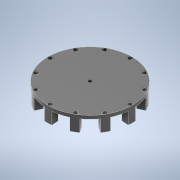
# Autodesk Inventor part: Platform
Saved by Autodesk Inventor 2022 (Build 260153000, 153)
## iProperties
Created: 2022-02-20
Part Number: Platform
Material: Genérico
Document SubType Name: Modeling
Designer: JK
Density: 1 g/cm^3
Appearance: Suave - Negro
Author: JK
Autodesk Inventor part; units mm, degrees
ref_plane "YZ Plane" through (0, 0, 0) normal (1, 0, 0) x (0, 1, 0)
ref_plane "XZ Plane" through (0, 0, 0) normal (0, 1, 0) x (-1, 0, 0)
ref_plane "XY Plane" through (0, 0, 0) normal (0, 0, 1) x (1, 0, 0)
sketch "Boceto1" plane through (0, 0, 0) normal (0, 1, 0) x (-1, 0, 0)
  circle A0 centre (0, 0) radius 62.862
  circle A1 centre (0, 0) radius 52.5
  dimension "d0" = 125.724
  dimension "d1" = 105
  constraints: 2 centre point, 2 coincident
  measures "d0" diameter of A0
  measures "d1" diameter of A1
extrude "Extrusión1" add sketch "Boceto1" along normal blind 23
sketch "Boceto2" plane through (0, 23, 0) normal (0, 1, 0) x (1, 0, 0)
  circle A0 centre (0, 0) radius 52.5 projected
extrude "Extrusión2" add sketch "Boceto2" against normal blind 5
sketch "Boceto3" plane through (0, 23, 0) normal (0, 1, 0) x (1, 0, 0)
  circle A0 centre (0, 0) radius 2.65
  dimension "d6" = 5.3
  constraints: 1 centre point, 1 coincident
  measures "d6" diameter of A0
extrude "Extrusión3" cut sketch "Boceto3" against normal through all
sketch "Boceto4" plane through (0, 23, 0) normal (0, 1, 0) x (1, 0, 0)
  circle A0 centre (-59.612, 0) radius 1.65
  point P0 (0, 0)
  dimension "d9" = 3.3
  dimension "d10" = 59.612
  constraints: 1 centre point
  measures "d9" diameter of A0
  measures "d10" distance of A0.centre point (0, 0)
extrude "Extrusión4" cut sketch "Boceto4" against normal through all
pattern_circular "Patrón circular1" count 12 over 360 about axis through (0, 0, 0) along (0, 1, 0) of "Extrusión4"
fillet "Empalme1" radius 3 1 edges at (52.5, 18, 0)
sketch "Boceto6" plane through (0, 23, 0) normal (0, 1, 0) x (1, 0, 0)
  circle A0 centre (0, -59.612) radius 1.65 projected
  circle A1 centre (0, -59.612) radius 2.85
  line L0 (1.6454, -62.462) -> (-1.6454, -62.462)
  line L1 (-1.6454, -62.462) -> (-3.2909, -59.612)
  line L2 (-3.2909, -59.612) -> (-1.6454, -56.762)
  line L3 (-1.6454, -56.762) -> (1.6454, -56.762)
  line L4 (1.6454, -56.762) -> (3.2909, -59.612)
  line L5 (3.2909, -59.612) -> (1.6454, -62.462)
  point P0 (0, 0)
  dimension "d20" = 5.7
  constraints: 12 end point, 2 coincident, 1 centre point, 1 horizontal alignment, 1 tangent, 13 other
  measures "d20" diameter of A1
extrude "Extrusión6" cut sketch "Boceto6" against normal blind 5 contours A0 | A1 | A1 L4 L5 | A1 L3 L4 | L5 L0 A1 | A1 L2 L3 | L0 L1 A1 | A1 L1 L2
pattern_circular "Patrón circular2" count 12 over 360 about axis through (0, 0, 0) along (0, 1, 0) of "Extrusión6"
sketch "Boceto7" plane through (0, 0, 0) normal (0, -1, 0) x (1, 0, 0)
  line L0 (0, 0) -> (-67.2382, 47.1765)
  line L1 (-67.2382, 47.1765) -> (-46.5407, 66.6024)
  circle A0 centre (0, 0) radius 2.65 projected
  line L2 (-46.5407, 66.6024) -> (0, 0)
  line L3 (0, 0) -> (-86.5562, 0)
  line L4 (0, 0) -> (-56.8894, 56.8894)
  point P0 (-1.5179, 2.1722)
  point P1 (-2.1693, 1.5221)
  dimension "d26" = 20
  dimension "d28" = 45
  constraints: 10 end point, 1 horizontal, 1 midpoint
  measures "d26" angle of L2 L0
  measures "d28" angle of L3 L4
extrude "Extrusión7" cut sketch "Boceto7" against normal up to surface (18 mm away) contours L0 L1 L4 A0 | A0 L4 L1 L2
pattern_circular "Patrón circular3" count 12 over 360 about axis through (0, 0, 0) along (0, 1, 0) of "Extrusión7"
